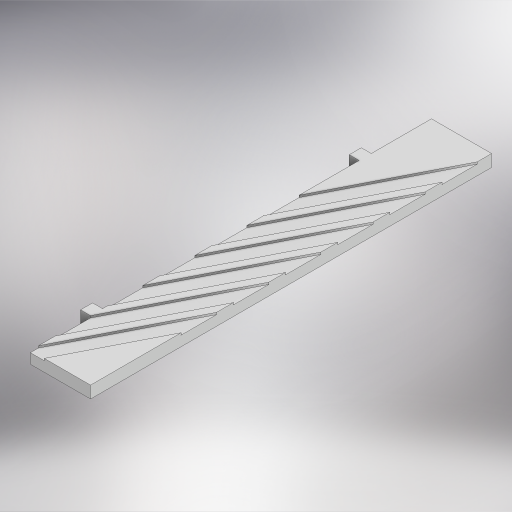
# Autodesk Inventor part: Module Cradle Right V1
Saved by Autodesk Inventor 2024 (Build 280153000, 153)
## iProperties
Created: 2024-03-20
Part Number: Module Cradle Right V1
Material: Generic
Document SubType Name: Modeling
Designer: cfang
Density: 1 g/cm^3
Appearance: Default
Author: cfang
Autodesk Inventor part; units mm, degrees
ref_plane "YZ Plane" through (0, 0, 0) normal (1, 0, 0) x (0, 1, 0)
ref_plane "XZ Plane" through (0, 0, 0) normal (0, 1, 0) x (-1, 0, 0)
ref_plane "XY Plane" through (0, 0, 0) normal (0, 0, 1) x (1, 0, 0)
sketch "Sketch3" plane through (0, 0, 0) normal (0, 1, 0) x (-1, 0, 0)
  line L0 (-15, -100) -> (15, -100)
  line L1 (15, -100) -> (15, 100)
  line L2 (15, 100) -> (-15, 100)
  line L3 (-15, 100) -> (-15, -100)
  line L4 (-15, -100) -> (15, 100) construction
  line L5 (15, -100) -> (-15, 100) construction
  point P0 (0, 0)
  dimension "d7" = 30
  dimension "d8" = 200
  constraints: 12 end point, 2 midpoint, 2 parallel, 1 horizontal, 1 perpendicular
  measures "d7" distance of L1.end L2.end
  measures "d8" distance of L0.end L1.end
extrude "Extrusion2" add sketch "Sketch3" along normal blind 6
sketch "Sketch5" plane through (0, 6, 0) normal (0, 1, 0) x (1, 0, 0)
  line L0 (-15, 100) -> (-15, -100) projected
  line L1 (-15, -113.6215) -> (15, -54.7432)
  line L2 (15, -100) -> (15, 100) projected
  line L3 (-15, -96) -> (15, -37.1217)
  line L4 (-15, -100) -> (15, -100) projected
  line L5 (-15, -70) -> (15, -11.1217)
  line L6 (-15, -87.6215) -> (15, -28.7432)
  line L7 (-15, -44) -> (15, 14.8783)
  line L8 (-15, -61.6215) -> (15, -2.7432)
  line L9 (-15, -18) -> (15, 40.8783)
  line L10 (-15, -35.6215) -> (15, 23.2568)
  line L11 (-15, 8) -> (15, 66.8783)
  line L12 (-15, -9.6215) -> (15, 49.2568)
  line L13 (-15, 34) -> (15, 92.8783)
  line L14 (-15, 16.3785) -> (15, 75.2568)
  point P0 (0, 0)
  point P1 (-8.0595, -100)
  point P2 (15, 75.2568)
  point P3 (15, 92.8783)
  point P4 (15, 49.2568)
  point P5 (15, 66.8783)
  point P6 (15, 23.2568)
  point P7 (15, 40.8783)
  point P8 (15, -2.7432)
  point P9 (15, 14.8783)
  point P10 (15, -28.7432)
  point P11 (15, -11.1217)
  dimension "d23" = 27
  dimension "d25" = 8
  dimension "d35" = 4
  dimension "d38" = 26
  constraints: 24 end point, 4 point on line, 1 parallel, 1 vertical, 30 other
  measures "d23" angle of L0 L1
  measures "d25" distance between parallel lines of L1 L3
  measures "d35" distance from line of L4 L3.start
  measures "d38" distance of L3.start L5.start
extrude "Extrusion4" cut sketch "Sketch5" against normal blind 1 contours L13 L2 L14 L0 | L11 L2 L12 L0 | L9 L2 L10 L0 | L7 L2 L8 L0 | L5 L2 L6 L0 | L3 L2 L1 L4 L0
sketch "Sketch6" plane through (-15, 0, -100) normal (-1, 0, 0) x (0, 0, 1)
  line L0 (0, 0) -> (200, 0) projected
  line L1 (0, 6) -> (66, 6) projected
  line L2 (30, 0) -> (36, 0)
  line L3 (36, 0) -> (36, 6)
  line L4 (36, 6) -> (30, 6)
  line L5 (30, 6) -> (30, 0)
  line L6 (164, 0) -> (170, 0)
  line L7 (170, 0) -> (170, 6)
  line L8 (170, 6) -> (164, 6)
  line L9 (164, 6) -> (164, 0)
  point P0 (100, 0)
  point P1 (100, 0)
  point P2 (164, 3)
  point P3 (100, 0)
  point P4 (30, 6)
  point P5 (36, 0)
  dimension "d43" = 6
  dimension "d44" = 6
  dimension "d45" = 64
  dimension "d46" = 64
  constraints: 16 end point, 4 parallel, 4 point on line, 3 midpoint, 2 horizontal, 2 perpendicular
  measures "d43" distance of L4.end L3.end
  measures "d44" distance of L8.end L7.end
  measures "d45" distance from line of L3 point (100, 0)
  measures "d46" horizontal distance of point (164, 3) point (100, 0)
extrude "Extrusion5" add sketch "Sketch6" along normal blind 5
equation "\"d46\" = d45"
body "Solid2"
